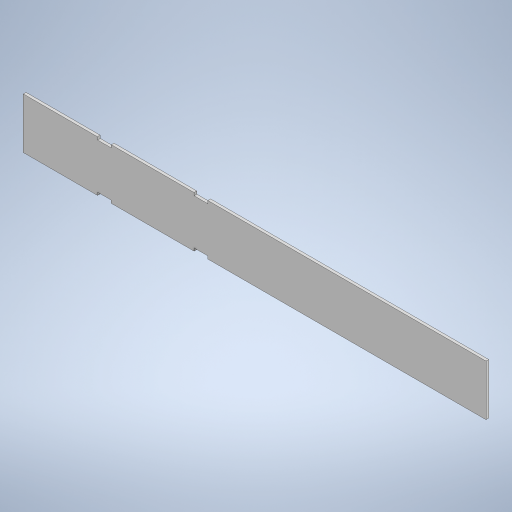
# Autodesk Inventor part: New base
Saved by Autodesk Inventor 2024 (Build 280153000, 153)
## iProperties
Created: 2023-07-10
Part Number: New base
Material: Generic
Document SubType Name: Modeling
Designer: USER
Density: 1 g/cm^3
Appearance: Default
Author: USER
Autodesk Inventor part; units mm, degrees
ref_plane "YZ Plane" through (0, 0, 0) normal (1, 0, 0) x (0, 1, 0)
ref_plane "XZ Plane" through (0, 0, 0) normal (0, 1, 0) x (-1, 0, 0)
ref_plane "XY Plane" through (0, 0, 0) normal (0, 0, 1) x (1, 0, 0)
sketch "Sketch1" plane through (0, 0, 0) normal (0, 0, 1) x (1, 0, 0)
  line L0 (86.5491, 25.4876) -> (86.5491, 28.0676)
  line L1 (86.5491, 28.0676) -> (86.5491, 25.4876)
  line L2 (73.8491, 25.4876) -> (86.5491, 25.4876)
  line L3 (86.5491, 25.4876) -> (73.8491, 25.4876)
  line L4 (86.5491, 28.0676) -> (217.6691, 28.0676)
  line L5 (217.6691, 28.0676) -> (86.5491, 28.0676)
  line L6 (217.6691, 28.0676) -> (217.6691, -18.6554)
  line L7 (217.6691, -18.6554) -> (217.6691, 28.0676)
  line L8 (86.5491, -18.6554) -> (217.6691, -18.6554)
  line L9 (217.6691, -18.6554) -> (86.5491, -18.6554)
  line L10 (-230.8205, -18.6554) -> (-230.8205, 28.0676)
  line L11 (-230.8205, 28.0676) -> (-230.8205, -18.6554)
  line L12 (-230.8205, 28.0676) -> (-230.8205, -18.6554)
  line L13 (-230.8205, -18.6554) -> (-230.8205, 28.0676)
  line L14 (-15.0509, -16.0754) -> (-15.0509, -18.6554)
  line L15 (-15.0509, -18.6554) -> (-15.0509, -16.0754)
  line L16 (-2.3509, 25.4876) -> (-2.3509, 28.0676)
  line L17 (-2.3509, 28.0676) -> (-2.3509, 25.4876)
  line L18 (-15.0509, 25.4876) -> (-2.3509, 25.4876)
  line L19 (-2.3509, 25.4876) -> (-15.0509, 25.4876)
  line L20 (-15.0509, 28.0676) -> (-15.0509, 25.4876)
  line L21 (-15.0509, 25.4876) -> (-15.0509, 28.0676)
  line L22 (-2.3509, -16.0754) -> (-15.0509, -16.0754)
  line L23 (-15.0509, -16.0754) -> (-2.3509, -16.0754)
  line L24 (-15.0509, 25.4876) -> (-15.0509, 28.0676)
  line L25 (-15.0509, 28.0676) -> (-15.0509, 25.4876)
  line L26 (-15.0509, -18.6554) -> (-15.0509, -16.0754)
  line L27 (-15.0509, -16.0754) -> (-15.0509, -18.6554)
  line L28 (-2.3509, 25.4876) -> (-15.0509, 25.4876)
  line L29 (-15.0509, 25.4876) -> (-2.3509, 25.4876)
  line L30 (-15.0509, -16.0754) -> (-2.3509, -16.0754)
  line L31 (-2.3509, -16.0754) -> (-15.0509, -16.0754)
  line L32 (-230.8205, 28.0676) -> (-15.0509, 28.0676)
  line L33 (-15.0509, 28.0676) -> (-230.8205, 28.0676)
  line L34 (-15.0509, 28.0676) -> (-230.8205, 28.0676)
  line L35 (-230.8205, 28.0676) -> (-15.0509, 28.0676)
  line L36 (-230.8205, -18.6554) -> (-15.0509, -18.6554)
  line L37 (-230.8205, -18.6554) -> (-15.0509, -18.6554)
  line L38 (-15.0509, -18.6554) -> (-230.8205, -18.6554)
  line L39 (-15.0509, -18.6554) -> (-230.8205, -18.6554)
  line L40 (-2.3509, -18.6554) -> (-2.3509, -16.0754)
  line L41 (73.8491, 28.0676) -> (73.8491, 25.4876)
  line L42 (73.8491, 25.4876) -> (73.8491, 28.0676)
  line L43 (-2.3509, 28.0676) -> (73.8491, 28.0676)
  line L44 (73.8491, 28.0676) -> (-2.3509, 28.0676)
  line L45 (86.5491, -18.6554) -> (86.5491, -16.0754)
  line L46 (86.5491, -16.0754) -> (86.5491, -18.6554)
  line L47 (86.5491, -16.0754) -> (73.8491, -16.0754)
  line L48 (73.8491, -16.0754) -> (86.5491, -16.0754)
  line L49 (-2.3509, -16.0754) -> (-2.3509, -18.6554)
  line L50 (-2.3509, 28.0676) -> (-2.3509, 25.4876)
  line L51 (-2.3509, 25.4876) -> (-2.3509, 28.0676)
  line L52 (-2.3509, -16.0754) -> (-2.3509, -18.6554)
  line L53 (-2.3509, -18.6554) -> (-2.3509, -16.0754)
  line L54 (73.8491, -18.6554) -> (-2.3509, -18.6554)
  line L55 (-2.3509, -18.6554) -> (73.8491, -18.6554)
  line L56 (-2.3509, -18.6554) -> (73.8491, -18.6554)
  line L57 (73.8491, -18.6554) -> (-2.3509, -18.6554)
  line L58 (73.8491, 28.0676) -> (-2.3509, 28.0676)
  line L59 (-2.3509, 28.0676) -> (73.8491, 28.0676)
  line L60 (73.8491, -16.0754) -> (73.8491, -18.6554)
  line L61 (73.8491, -18.6554) -> (73.8491, -16.0754)
  line L62 (73.8491, -18.6554) -> (73.8491, -16.0754)
  line L63 (73.8491, -16.0754) -> (73.8491, -18.6554)
  line L64 (73.8491, -16.0754) -> (86.5491, -16.0754)
  line L65 (86.5491, -16.0754) -> (73.8491, -16.0754)
  line L66 (86.5491, 25.4876) -> (73.8491, 25.4876)
  line L67 (73.8491, 25.4876) -> (86.5491, 25.4876)
  line L68 (73.8491, 25.4876) -> (73.8491, 28.0676)
  line L69 (73.8491, 28.0676) -> (73.8491, 25.4876)
  line L70 (86.5491, -16.0754) -> (86.5491, -18.6554)
  line L71 (86.5491, -18.6554) -> (86.5491, -16.0754)
  line L72 (217.6691, 28.0676) -> (86.5491, 28.0676)
  line L73 (86.5491, 28.0676) -> (217.6691, 28.0676)
  line L74 (217.6691, -18.6554) -> (217.6691, 28.0676)
  line L75 (217.6691, 28.0676) -> (217.6691, -18.6554)
  line L76 (86.5491, 28.0676) -> (86.5491, 25.4876)
  line L77 (86.5491, 25.4876) -> (86.5491, 28.0676)
  line L78 (86.5491, -18.6554) -> (217.6691, -18.6554)
  line L79 (217.6691, -18.6554) -> (86.5491, -18.6554)
  point P0 (0, 0)
  constraints: 158 end point, 3 other
extrude "Extrusion1" add sketch "Sketch1" along normal blind 2.5
move faces "Move1" translate (23, 0, 0) faces at (217.6691, -3.081, 0.8333)
move faces "Move2" translate (2, 0, 0) faces at (240.6691, 12.4933, 1.6667)
sketch "Sketch2" plane through (0, 0, 2.5) normal (0, 0, 1) x (1, 0, 0)
  line L0 (-83.3964, 28.0676) -> (-230.8205, 28.0676)
  line L1 (-230.8205, 28.0676) -> (-230.8205, -18.6554)
  line L2 (-230.8205, -18.6554) -> (-83.3964, -18.6554)
  line L3 (-83.3964, -18.6554) -> (-83.3964, 28.0676)
  constraints: 8 end point, 2 parallel, 1 horizontal, 1 perpendicular
extrude "Extrusion2" cut sketch "Sketch2" against normal blind 10
sketch "Sketch4" plane through (-83.3964, -18.6554, 2.5) normal (-1, 0, 0) x (0, 0, 1)
  line L0 (-2.5, 0) -> (-2.5, 46.723) projected
  line L1 (-2.5, 46.723) -> (0, 46.723) projected
  line L2 (0, 46.723) -> (0, 0) projected
  line L3 (0, 0) -> (-2.5, 0) projected
  point P0 (-2.5, 18.6554)
extrude "Extrusion3" add sketch "Sketch4" along normal blind 75
sketch "Sketch5" plane through (242.6691, -18.6554, 0) normal (1, 0, 0) x (0, 0, -1)
  line L0 (-2.5, 0) -> (-2.5, 46.723) projected
  line L1 (0, 46.723) -> (-2.5, 46.723) projected
  line L2 (0, 0) -> (0, 46.723) projected
  line L3 (0, 0) -> (-2.5, 0) projected
  point P0 (0, 18.6554)
extrude "Extrusion4" add sketch "Sketch5" along normal blind 100
sketch "Sketch6" plane through (-158.3964, -18.6554, 2.5) normal (-1, 0, 0) x (0, 0, 1)
  line L0 (-2.5, 46.723) -> (-2.5, 0) projected
  line L1 (0, 0) -> (0, 46.723) projected
  line L2 (0, 46.723) -> (-2.5, 46.723) projected
  line L3 (-2.5, 0) -> (0, 0) projected
  point P0 (-2.5, 18.6554)
extrude "Extrusion5" cut sketch "Sketch6" against normal blind 75
body "Solid1"
